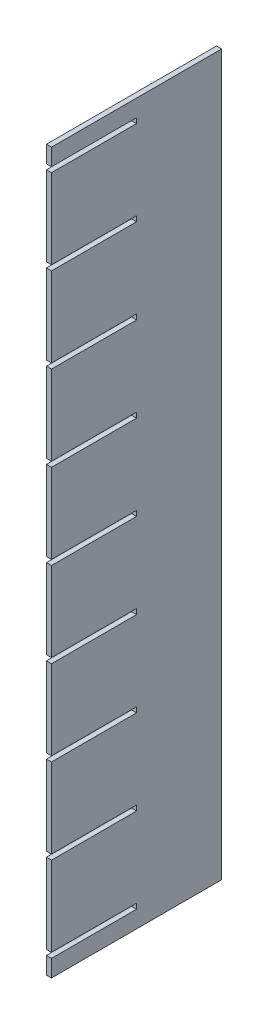
# Autodesk Inventor part: Separators
Saved by Autodesk Inventor 2024 (Build 280153000, 153)
## iProperties
Created: 2023-07-19
Part Number: Separators
Material: Generic
Document SubType Name: Modeling
Designer: Bruno
Density: 1 g/cm^3
Appearance: Default
Author: Bruno
Autodesk Inventor part; units mm, degrees
ref_plane "YZ Plane" through (0, 0, 0) normal (1, 0, 0) x (0, 1, 0)
ref_plane "XZ Plane" through (0, 0, 0) normal (0, 1, 0) x (-1, 0, 0)
ref_plane "XY Plane" through (0, 0, 0) normal (0, 0, 1) x (1, 0, 0)
sketch "Sketch1" plane through (0, 0, 0) normal (1, 0, 0) x (0, 1, 0)
  line L0 (-13, 100) -> (-59.9, 100)
  line L1 (-13, 100) -> (-13, 50)
  line L2 (-59.9, 100) -> (-59.9, 50)
  line L3 (-59.9, 50) -> (-63, 50)
  line L4 (-63, 50) -> (-63, 100)
  line L5 (-10, 50) -> (-10, 100)
  line L6 (-10, 100) -> (0, 100)
  line L7 (0, 100) -> (0, 0)
  line L8 (-10, 50) -> (-13, 50)
  line L9 (-63, 100) -> (-109.9, 100)
  line L10 (-109.9, 50) -> (-113, 50)
  line L11 (-109.9, 100) -> (-109.9, 50)
  line L12 (-113, 50) -> (-113, 100)
  line L13 (-113, 100) -> (-159.9, 100)
  line L14 (-159.9, 50) -> (-163, 50)
  line L15 (-159.9, 100) -> (-159.9, 50)
  line L16 (-163, 50) -> (-163, 100)
  line L17 (-163, 100) -> (-209.9, 100)
  line L18 (-209.9, 50) -> (-213, 50)
  line L19 (-209.9, 100) -> (-209.9, 50)
  line L20 (-213, 50) -> (-213, 100)
  line L21 (-213, 100) -> (-259.9, 100)
  line L22 (-259.9, 50) -> (-263, 50)
  line L23 (-259.9, 100) -> (-259.9, 50)
  line L24 (-263, 50) -> (-263, 100)
  line L25 (-263, 100) -> (-309.9, 100)
  line L26 (-309.9, 50) -> (-313, 50)
  line L27 (-309.9, 100) -> (-309.9, 50)
  line L28 (-313, 50) -> (-313, 100)
  line L29 (-313, 100) -> (-359.9, 100)
  line L30 (-359.9, 50) -> (-363, 50)
  line L31 (-359.9, 100) -> (-359.9, 50)
  line L32 (-363, 50) -> (-363, 100)
  line L33 (-363, 100) -> (-409.9, 100)
  line L34 (-409.9, 50) -> (-413, 50)
  line L35 (-409.9, 100) -> (-409.9, 50)
  line L36 (-413, 50) -> (-413, 100)
  line L37 (-413, 100) -> (-423, 100)
  line L38 (-423, 100) -> (-423, 0)
  line L39 (-423, 0) -> (0, 0)
  point P0 (-11.5, 50)
  dimension "d4" = 3.1
  dimension "d5" = 3
  dimension "d6" = 10
  dimension "d7" = 100
  dimension "d8" = 50
  dimension "d11" = 50
  dimension "d16" = 10
  constraints: 80 end point, 5 horizontal, 4 perpendicular, 4 vertical, 3 parallel, 2 coincident, 1 collinear, 1 midpoint, 62 other
  measures "d4" distance of L2.end L3.end
  measures "d5" distance of L1.end L5.start
  measures "d6" distance of L5.end L6.end
  measures "d7" distance of L6.end L7.end
  measures "d8" vertical distance of L7.end point (-11.5, 50)
  measures "d11" distance of L0.end L9.end
  measures "d16" distance of L36.end L37.end
extrude "Extrusion1" add sketch "Sketch1" along normal blind 3
body "Solid1"
